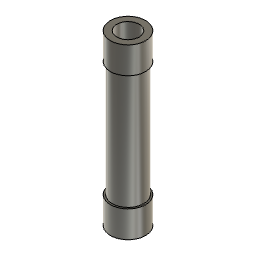
ベアリング内ネジ v1 (Autodesk Fusion 360 design; units mm, degrees)
Autodesk Fusion 360 part; units mm, degrees
sketch "スケッチ17" plane through (0, 0, 0) normal (0, 0, 1) x (1, 0, 0)
  circle A0 centre (0, 0) radius 2.5
  dimension "d50" = 5
  constraint coincident A0.centre origin
  measures "d50" diameter of A0
extrude "押し出し14" add sketch "スケッチ17" along normal blind 3.8
sketch "スケッチ18" plane through (0, 0, 3.8) normal (0, 0, 1) x (-1, 0, 0)
  circle A0 centre (0, 0) radius 2.5
  circle A1 centre (0, 0) radius 2.25
  dimension "d53" = 4.5
  constraint concentric A0 A1
  measures "d53" diameter of A1
extrude "押し出し15" add sketch "スケッチ18" along normal blind 16.4 contours A1
sketch "スケッチ19" plane through (0, 0, 20.2) normal (0, 0, 1) x (-1, 0, 0)
  circle A0 centre (0, 0) radius 2.25
  circle A1 centre (0, 0) radius 2.5
  dimension "d56" = 5
  constraint coincident A0.centre A1.centre
  measures "d56" diameter of A1
extrude "押し出し16" add sketch "スケッチ19" along normal blind 3.8 contours A0 | A1
sketch "スケッチ20" plane through (0, 0, 24) normal (0, 0, 1) x (-1, 0, 0)
  circle A0 centre (0, 0) radius 2.5
  circle A1 centre (0, 0) radius 1.585
  dimension "d59" = 3.17
  constraint concentric A0 A1
  measures "d59" diameter of A1
extrude "押し出し17" cut sketch "スケッチ20" against normal blind 24 contours A1
